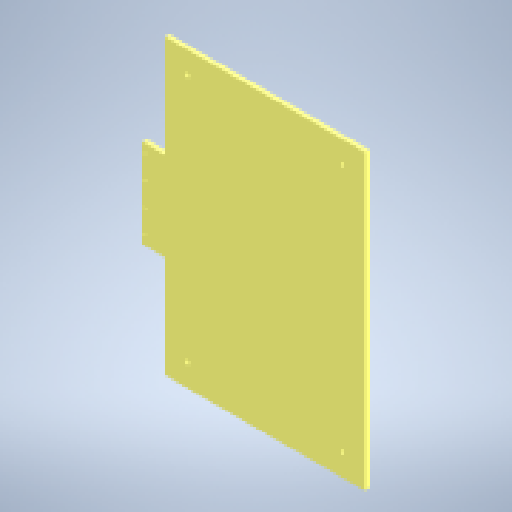
# Autodesk Inventor part: base
Saved by Autodesk Inventor 2024 (Build 280153000, 153)
## iProperties
Created: 2023-12-23
Part Number: base
Material: Generico
Document SubType Name: Modeling
Designer: Giorgio
Density: 1 g/cm^3
Appearance: Default
Mass: 2700 g
Surface Area: 5610 cm^2
Volume: 2700 cm^3
Author: Giorgio
Autodesk Inventor part; units mm, degrees
ref_plane "YZ Plane" through (0, 0, 0) normal (1, 0, 0) x (0, 1, 0)
ref_plane "XZ Plane" through (0, 0, 0) normal (0, 1, 0) x (-1, 0, 0)
ref_plane "XY Plane" through (0, 0, 0) normal (0, 0, 1) x (1, 0, 0)
sketch "Schizzo1" plane through (0, 0, 0) normal (0, 0, 1) x (1, 0, 0)
  line L0 (-225, 330) -> (225, 330)
  line L1 (225, 330) -> (225, -330)
  line L2 (225, -330) -> (-225, -330)
  line L3 (-225, -50) -> (-275, -50)
  line L4 (-275, -50) -> (-275, 50)
  line L5 (-275, 50) -> (-225, 50)
  line L6 (-225, -330) -> (-225, -50)
  line L7 (-225, 50) -> (-225, 330)
  circle A0 centre (-88.8619, 71.07) radius 2.5
  point P0 (0, 0)
  point P1 (0, 330)
  dimension "d0" = 450
  dimension "d1" = 660
  dimension "d4" = 100
  dimension "d5" = 280
  dimension "d7" = 225
  dimension "d50" = 5
  dimension "d51" = 330
  constraints: 16 end point, 4 parallel, 2 horizontal, 2 perpendicular, 1 centre point, 1 midpoint
  measures "d0" distance of L0.start L0.end
  measures "d1" distance of L0.end L1.end
  measures "d4" distance of L3.end L4.end
  measures "d5" distance between parallel lines of L3 L2
  measures "d7" distance from line of point (0, 0) L1
  measures "d50" diameter of A0
  measures "d51" distance of point (0, 330) point (0, 0)
extrude "Estrusione1" add sketch "Schizzo1" along normal blind 10 contours L0 L1 L2 L6 L3 L4 L5 L7 | A0
sketch "Schizzo2" plane through (0, 0, 10) normal (0, 0, 1) x (1, 0, 0)
  circle A0 centre (-175, 280) radius 4.25
  circle A1 centre (175, 280) radius 4.25
  circle A2 centre (175, -280) radius 4.25
  circle A3 centre (-175, -280) radius 4.25
  line L0 (225, -330) -> (225, 330) projected
  line L1 (-225, 330) -> (-225, 50) projected
  line L2 (-225, -50) -> (-225, -330) projected
  line L3 (-225, -330) -> (225, -330) projected
  line L4 (225, 330) -> (-225, 330) projected
  circle A4 centre (-270, 30) radius 2
  circle A5 centre (-270, -30) radius 2
  line L5 (-275, 50) -> (-275, -50) projected
  line L6 (-225, 50) -> (-275, 50) projected
  line L7 (-275, -50) -> (-225, -50) projected
  circle A6 centre (-150, 60) radius 2.75
  circle A7 centre (0, 60) radius 2.75
  circle A8 centre (150, 60) radius 2.75
  circle A9 centre (-150, 90) radius 2.75
  circle A10 centre (0, 90) radius 2.75
  circle A11 centre (150, 90) radius 2.75
  circle A12 centre (-150, -90) radius 2.75
  circle A13 centre (0, -90) radius 2.75
  circle A14 centre (150, -90) radius 2.75
  circle A15 centre (-150, -60) radius 2.75
  circle A16 centre (0, -60) radius 2.75
  circle A17 centre (150, -60) radius 2.75
  circle A18 centre (-260, -45) radius 2
  circle A19 centre (-260, 45) radius 2
  circle A20 centre (-235, 45) radius 2
  circle A21 centre (-235, -45) radius 2
  point P0 (0, 0)
  dimension "d8" = 50
  dimension "d9" = 50
  dimension "d10" = 50
  dimension "d11" = 50
  dimension "d12" = 50
  dimension "d13" = 50
  dimension "d14" = 50
  dimension "d15" = 50
  dimension "d16" = 8.5
  dimension "d17" = 8.5
  dimension "d18" = 8.5
  dimension "d19" = 8.5
  dimension "d20" = 5
  dimension "d23" = 5
  dimension "d24" = 4
  dimension "d27" = 4
  dimension "d28" = 20
  dimension "d29" = 20
  dimension "d49" = 450
  dimension "d52" = 5.5
  dimension "d55" = 150
  dimension "d58" = 30
  dimension "d61" = 0
  dimension "d62" = 60
  dimension "d63" = 5.5
  dimension "d66" = 150
  dimension "d69" = 30
  dimension "d72" = 0
  dimension "d73" = 60
  dimension "d74" = 4
  dimension "d78" = 90
  dimension "d86" = 25
  dimension "d92" = 5
  dimension "d93" = 10
  constraints: 22 centre point, 3 horizontal, 3 vertical, 26 other
  measures "d8" distance from line of L0 A1.centre
  measures "d9" distance from line of L0 A2.centre
  measures "d10" distance from line of L1 A0.centre
  measures "d11" distance from line of L2 A3.centre
  measures "d12" distance from line of L3 A2.centre
  measures "d13" distance from line of L4 A1.centre
  measures "d14" distance from line of L4 A0.centre
  measures "d15" distance from line of L3 A3.centre
  measures "d16" diameter of A3
  measures "d17" diameter of A2
  measures "d18" diameter of A1
  measures "d19" diameter of A0
  measures "d20" distance from line of L5 A4.centre
  measures "d23" distance from line of L5 A5.centre
  measures "d24" diameter of A4
  measures "d27" diameter of A5
  measures "d28" distance from line of A4.centre L6
  measures "d29" distance from line of L7 A5.centre
  measures "d49" distance between parallel lines of L1 L0
  measures "d52" diameter of A6
  measures "d55" distance of A6.centre A7.centre
  measures "d58" distance of A6.centre A9.centre
  measures "d61" horizontal distance of A7.centre point (0, 0)
  measures "d62" distance of point (0, 0) A7.centre
  measures "d63" diameter of A12
  measures "d66" distance of A12.centre A13.centre
  measures "d69" distance of A12.centre A15.centre
  measures "d72" horizontal distance of point (0, 0) A16.centre
  measures "d73" distance of point (0, 0) A16.centre
  measures "d74" diameter of A18
  measures "d78" distance of A18.centre A19.centre
  measures "d86" distance of A19.centre A20.centre
  measures "d92" distance from line of A20.centre L6
  measures "d93" horizontal distance of A4.centre A19.centre
extrude "Estrusione2" cut sketch "Schizzo2" against normal blind 10 contours A0 | A1 | A2 | A3 | A4 | A5 | A6 | A7 | A8 | A9 | A10 | A11 | A12 | A13 | A14 | A15 | A16 | A17 | A18 | A19 | A20 | A21
equation "\"d5\" = -0.5 * d4 + 0.5 * d1"
equation "\"d7\" = 0.5 * d0"
equation "\"d51\" = 0.5 * d1"
equation "\"d9\" = d8"
equation "\"d10\" = d8"
equation "\"d11\" = d8"
equation "\"d12\" = d8"
equation "\"d13\" = d8"
equation "\"d14\" = d10"
equation "\"d15\" = d8"
equation "\"d17\" = d16"
equation "\"d18\" = d16"
equation "\"d19\" = d16"
equation "\"d23\" = d20"
equation "\"d27\" = d24"
